Autodesk Fusion 360 part; units mm, degrees
(part 7 of 8)
  line L1736 (-325.3503, 148.8501) -> (-322.3503, 148.8501)
  line L1737 (-322.3503, 148.8501) -> (-322.3503, 151.8501)
  line L1738 (-322.3503, 151.8501) -> (-325.3503, 151.8501)
  line L1739 (-325.3503, 151.8501) -> (-325.3503, 154.8501)
  line L1740 (-325.3503, 154.8501) -> (-322.3503, 154.8501)
  line L1741 (-322.3503, 154.8501) -> (-322.3503, 157.8501)
  line L1742 (-322.3503, 157.8501) -> (-325.3503, 157.8501)
  line L1743 (-325.3503, 157.8501) -> (-325.3503, 160.8501)
  line L1744 (-325.3503, 160.8501) -> (-322.3503, 160.8501)
  line L1745 (-322.3503, 160.8501) -> (-322.3503, 163.8501)
  line L1746 (-322.3503, 163.8501) -> (-325.3503, 163.8501)
  line L1747 (-325.3503, 163.8501) -> (-325.3503, 166.8501)
  line L1748 (-325.3503, 166.8501) -> (-322.3503, 166.8501)
  line L1749 (-322.3503, 166.8501) -> (-322.3503, 169.8501)
  line L1750 (-322.3503, 169.8501) -> (-325.3503, 169.8501)
  line L1751 (-325.3503, 169.8501) -> (-325.3503, 172.8501)
  line L1752 (-325.3503, 172.8501) -> (-322.3503, 172.8501)
  line L1753 (-322.3503, 172.8501) -> (-322.3503, 176.6001)
  line L1754 (-322.3503, 176.6001) -> (-325.3503, 176.6001)
  line L1755 (-325.3503, 176.6001) -> (-325.3503, 177.3501)
  line L1756 (-325.3503, 177.3501) -> (-327.1003, 177.3501)
  line L1757 (-327.1003, 177.3501) -> (-327.1003, 180.3501)
  line L1758 (-327.1003, 180.3501) -> (-331.8503, 180.3501)
  line L1759 (-331.8503, 180.3501) -> (-331.8503, 177.3501)
  line L1760 (-331.8503, 177.3501) -> (-334.8503, 177.3501)
  line L1761 (-334.8503, 177.3501) -> (-334.8503, 180.3501)
  line L1762 (-334.8503, 180.3501) -> (-337.8503, 180.3501)
  line L1763 (-337.8503, 180.3501) -> (-337.8503, 177.3501)
  line L1764 (-337.8503, 177.3501) -> (-340.8503, 177.3501)
  line L1765 (-340.8503, 177.3501) -> (-340.8503, 180.3501)
  line L1766 (-340.8503, 180.3501) -> (-343.8503, 180.3501)
  line L1767 (-343.8503, 180.3501) -> (-343.8503, 177.3501)
  line L1768 (-343.8503, 177.3501) -> (-346.8503, 177.3501)
  line L1769 (-346.8503, 177.3501) -> (-346.8503, 180.3501)
  line L1770 (-346.8503, 180.3501) -> (-349.8503, 180.3501)
  line L1771 (-349.8503, 180.3501) -> (-349.8503, 177.3501)
  line L1772 (-349.8503, 177.3501) -> (-352.8503, 177.3501)
  line L1773 (-352.8503, 177.3501) -> (-352.8503, 180.3501)
  line L1774 (-352.8503, 180.3501) -> (-355.8503, 180.3501)
  line L1775 (-355.8503, 180.3501) -> (-355.8503, 177.3501)
  line L1776 (-355.8503, 177.3501) -> (-358.8503, 177.3501)
  line L1777 (-358.8503, 177.3501) -> (-358.8503, 180.3501)
  line L1778 (-358.8503, 180.3501) -> (-361.8503, 180.3501)
  line L1779 (-361.8503, 180.3501) -> (-361.8503, 177.3501)
  line L1780 (-361.8503, 177.3501) -> (-364.8503, 177.3501)
  line L1781 (-364.8503, 177.3501) -> (-364.8503, 180.3501)
  line L1782 (-364.8503, 180.3501) -> (-367.8503, 180.3501)
  line L1783 (-367.8503, 180.3501) -> (-367.8503, 177.3501)
  line L1784 (-367.8503, 177.3501) -> (-370.8503, 177.3501)
  line L1785 (-370.8503, 177.3501) -> (-370.8503, 180.3501)
  line L1786 (-370.8503, 180.3501) -> (-373.8503, 180.3501)
  line L1787 (-373.8503, 180.3501) -> (-373.8503, 177.3501)
  line L1788 (-373.8503, 177.3501) -> (-376.8503, 177.3501)
  line L1789 (-376.8503, 177.3501) -> (-376.8503, 180.3501)
  line L1790 (-376.8503, 180.3501) -> (-379.8503, 180.3501)
  line L1791 (-379.8503, 180.3501) -> (-379.8503, 177.3501)
  line L1792 (-379.8503, 177.3501) -> (-382.8503, 177.3501)
  line L1793 (-382.8503, 177.3501) -> (-382.8503, 180.3501)
  line L1794 (-382.8503, 180.3501) -> (-385.8503, 180.3501)
  line L1795 (-385.8503, 180.3501) -> (-385.8503, 177.3501)
  line L1796 (-385.8503, 177.3501) -> (-388.8503, 177.3501)
  line L1797 (-388.8503, 177.3501) -> (-388.8503, 180.3501)
  line L1798 (-388.8503, 180.3501) -> (-391.8503, 180.3501)
  line L1799 (-391.8503, 180.3501) -> (-391.8503, 177.3501)
  line L1800 (-391.8503, 177.3501) -> (-394.8503, 177.3501)
  line L1801 (-394.8503, 177.3501) -> (-394.8503, 180.3501)
  line L1802 (-394.8503, 180.3501) -> (-397.8503, 180.3501)
  line L1803 (-397.8503, 180.3501) -> (-397.8503, 177.3501)
  line L1804 (-397.8503, 177.3501) -> (-400.8503, 177.3501)
  line L1805 (-400.8503, 177.3501) -> (-400.8503, 180.3501)
  line L1806 (-400.8503, 180.3501) -> (-403.8503, 180.3501)
  line L1807 (-403.8503, 180.3501) -> (-403.8503, 177.3501)
  line L1808 (-403.8503, 177.3501) -> (-406.8503, 177.3501)
  line L1809 (-406.8503, 177.3501) -> (-406.8503, 180.3501)
  line L1810 (-406.8503, 180.3501) -> (-409.8503, 180.3501)
  line L1811 (-409.8503, 180.3501) -> (-409.8503, 177.3501)
  line L1812 (-409.8503, 177.3501) -> (-412.8503, 177.3501)
  line L1813 (-412.8503, 177.3501) -> (-412.8503, 180.3501)
  line L1814 (-412.8503, 180.3501) -> (-415.8503, 180.3501)
  line L1815 (-415.8503, 180.3501) -> (-415.8503, 177.3501)
  line L1816 (-415.8503, 177.3501) -> (-418.8503, 177.3501)
  line L1817 (-418.8503, 177.3501) -> (-418.8503, 180.3501)
  line L1818 (-418.8503, 180.3501) -> (-421.8503, 180.3501)
  line L1819 (-421.8503, 180.3501) -> (-421.8503, 177.3501)
  line L1820 (-421.8503, 177.3501) -> (-424.8503, 177.3501)
  line L1821 (-424.8503, 177.3501) -> (-424.8503, 180.3501)
  line L1822 (-424.8503, 180.3501) -> (-427.8504, 180.3501)
  line L1823 (-427.8504, 180.3501) -> (-427.8504, 177.3501)
  line L1824 (-427.8504, 177.3501) -> (-430.8504, 177.3501)
  line L1825 (-430.8504, 177.3501) -> (-430.8504, 180.3501)
  line L1826 (-430.8504, 180.3501) -> (-433.8504, 180.3501)
  line L1827 (-433.8504, 180.3501) -> (-433.8504, 177.3501)
  line L1828 (-433.8504, 177.3501) -> (-436.8504, 177.3501)
  line L1829 (-436.8504, 177.3501) -> (-436.8504, 180.3501)
  line L1830 (-436.8504, 180.3501) -> (-439.8504, 180.3501)
  line L1831 (-439.8504, 180.3501) -> (-439.8504, 177.3501)
  line L1832 (-439.8504, 177.3501) -> (-442.8504, 177.3501)
  line L1833 (-442.8504, 177.3501) -> (-442.8504, 180.3501)
  line L1834 (-442.8504, 180.3501) -> (-445.8504, 180.3501)
  line L1835 (-445.8504, 180.3501) -> (-445.8504, 177.3501)
  line L1836 (-445.8504, 177.3501) -> (-448.8504, 177.3501)
  line L1837 (-448.8504, 177.3501) -> (-448.8504, 180.3501)
  line L1838 (-448.8504, 180.3501) -> (-451.8504, 180.3501)
  line L1839 (-451.8504, 180.3501) -> (-451.8504, 177.3501)
  line L1840 (-451.8504, 177.3501) -> (-454.8504, 177.3501)
  line L1841 (-454.8504, 177.3501) -> (-454.8504, 180.3501)
  line L1842 (-454.8504, 180.3501) -> (-457.8504, 180.3501)
  line L1843 (-457.8504, 180.3501) -> (-457.8504, 177.3501)
  line L1844 (-457.8504, 177.3501) -> (-460.8504, 177.3501)
  line L1845 (-460.8504, 177.3501) -> (-460.8504, 180.3501)
  line L1846 (-460.8504, 180.3501) -> (-463.8504, 180.3501)
  line L1847 (-463.8504, 180.3501) -> (-463.8504, 177.3501)
  line L1848 (-463.8504, 177.3501) -> (-466.8504, 177.3501)
  line L1849 (-466.8504, 177.3501) -> (-466.8504, 180.3501)
  line L1850 (-466.8504, 180.3501) -> (-469.8504, 180.3501)
  line L1851 (-469.8504, 180.3501) -> (-469.8504, 177.3501)
  line L1852 (-469.8504, 177.3501) -> (-472.8504, 177.3501)
  line L1853 (-472.8504, 177.3501) -> (-472.8504, 180.3501)
  line L1854 (-472.8504, 180.3501) -> (-475.8504, 180.3501)
  line L1855 (-475.8504, 180.3501) -> (-475.8504, 177.3501)
  line L1856 (-475.8504, 177.3501) -> (-478.8504, 177.3501)
  line L1857 (-478.8504, 177.3501) -> (-478.8504, 180.3501)
  line L1858 (-478.8504, 180.3501) -> (-481.8504, 180.3501)
  line L1859 (-481.8504, 180.3501) -> (-481.8504, 177.3501)
  line L1860 (-481.8504, 177.3501) -> (-484.8504, 177.3501)
  line L1861 (-484.8504, 177.3501) -> (-484.8504, 180.3501)
  line L1862 (-484.8504, 180.3501) -> (-487.8504, 180.3501)
  line L1863 (-487.8504, 180.3501) -> (-487.8504, 177.3501)
  line L1864 (-487.8504, 177.3501) -> (-490.8504, 177.3501)
  line L1865 (-490.8504, 177.3501) -> (-490.8504, 180.3501)
  line L1866 (-490.8504, 180.3501) -> (-493.8504, 180.3501)
  line L1867 (-493.8504, 180.3501) -> (-493.8504, 177.3501)
  line L1868 (-493.8504, 177.3501) -> (-496.8504, 177.3501)
  line L1869 (-496.8504, 177.3501) -> (-496.8504, 180.3501)
  line L1870 (-496.8504, 180.3501) -> (-499.8504, 180.3501)
  line L1871 (-499.8504, 180.3501) -> (-499.8504, 177.3501)
  line L1872 (-499.8504, 177.3501) -> (-502.8504, 177.3501)
  line L1873 (-502.8504, 177.3501) -> (-502.8504, 180.3501)
  line L1874 (-502.8504, 180.3501) -> (-505.8504, 180.3501)
  line L1875 (-505.8504, 180.3501) -> (-505.8504, 177.3501)
  line L1876 (-505.8504, 177.3501) -> (-508.8504, 177.3501)
  line L1877 (-508.8504, 177.3501) -> (-508.8504, 180.3501)
  line L1878 (-508.8504, 180.3501) -> (-511.8504, 180.3501)
  line L1879 (-511.8504, 180.3501) -> (-511.8504, 177.3501)
  line L1880 (-511.8504, 177.3501) -> (-514.8504, 177.3501)
  line L1881 (-514.8504, 177.3501) -> (-514.8504, 180.3501)
  line L1882 (-514.8504, 180.3501) -> (-517.8504, 180.3501)
  line L1883 (-517.8504, 180.3501) -> (-517.8504, 177.3501)
  line L1884 (-517.8504, 177.3501) -> (-520.8504, 177.3501)
  line L1885 (-520.8504, 177.3501) -> (-520.8504, 180.3501)
  line L1886 (-520.8504, 180.3501) -> (-523.8504, 180.3501)
  line L1887 (-523.8504, 180.3501) -> (-523.8504, 177.3501)
  line L1888 (-523.8504, 177.3501) -> (-526.8504, 177.3501)
  line L1889 (-526.8504, 177.3501) -> (-526.8504, 180.3501)
  line L1890 (-526.8504, 180.3501) -> (-529.8504, 180.3501)
  line L1891 (-529.8504, 180.3501) -> (-529.8504, 177.3501)
  line L1892 (-529.8504, 177.3501) -> (-532.8504, 177.3501)
  line L1893 (-532.8504, 177.3501) -> (-532.8504, 180.3501)
  line L1894 (-532.8504, 180.3501) -> (-535.8504, 180.3501)
  line L1895 (-535.8504, 180.3501) -> (-535.8504, 177.3501)
  line L1896 (-535.8504, 177.3501) -> (-538.8504, 177.3501)
  line L1897 (-538.8504, 177.3501) -> (-538.8504, 180.3501)
  line L1898 (-538.8504, 180.3501) -> (-541.8504, 180.3501)
  line L1899 (-541.8504, 180.3501) -> (-541.8504, 177.3501)
  line L1900 (-541.8504, 177.3501) -> (-544.8504, 177.3501)
  line L1901 (-544.8504, 177.3501) -> (-544.8504, 180.3501)
  line L1902 (-544.8504, 180.3501) -> (-547.8505, 180.3501)
  line L1903 (-547.8505, 180.3501) -> (-547.8505, 177.3501)
  line L1904 (-547.8505, 177.3501) -> (-550.8505, 177.3501)
  line L1905 (-550.8505, 177.3501) -> (-550.8505, 180.3501)
  line L1906 (-550.8505, 180.3501) -> (-553.8505, 180.3501)
  line L1907 (-553.8505, 180.3501) -> (-553.8505, 177.3501)
  line L1908 (-553.8505, 177.3501) -> (-556.8505, 177.3501)
  line L1909 (-556.8505, 177.3501) -> (-556.8505, 180.3501)
  line L1910 (-556.8505, 180.3501) -> (-559.8505, 180.3501)
  line L1911 (-559.8505, 180.3501) -> (-559.8505, 177.3501)
  line L1912 (-559.8505, 177.3501) -> (-562.8505, 177.3501)
  line L1913 (-562.8505, 177.3501) -> (-562.8505, 180.3501)
  line L1914 (-562.8505, 180.3501) -> (-565.8505, 180.3501)
  line L1915 (-565.8505, 180.3501) -> (-565.8505, 177.3501)
  line L1916 (-565.8505, 177.3501) -> (-568.8505, 177.3501)
  line L1917 (-568.8505, 177.3501) -> (-568.8505, 180.3501)
  line L1918 (-568.8505, 180.3501) -> (-571.8505, 180.3501)
  line L1919 (-571.8505, 180.3501) -> (-571.8505, 177.3501)
  line L1920 (-571.8505, 177.3501) -> (-574.8505, 177.3501)
  line L1921 (-574.8505, 177.3501) -> (-574.8505, 180.3501)
  line L1922 (-574.8505, 180.3501) -> (-577.8505, 180.3501)
  line L1923 (-577.8505, 180.3501) -> (-577.8505, 177.3501)
  line L1924 (-577.8505, 177.3501) -> (-580.8505, 177.3501)
  line L1925 (-580.8505, 177.3501) -> (-580.8505, 180.3501)
  line L1926 (-580.8505, 180.3501) -> (-583.8505, 180.3501)
  line L1927 (-583.8505, 180.3501) -> (-583.8505, 177.3501)
  line L1928 (-583.8505, 177.3501) -> (-586.8505, 177.3501)
  line L1929 (-586.8505, 177.3501) -> (-586.8505, 180.3501)
  line L1930 (-586.8505, 180.3501) -> (-589.8505, 180.3501)
  line L1931 (-589.8505, 180.3501) -> (-589.8505, 177.3501)
  line L1932 (-589.8505, 177.3501) -> (-592.8505, 177.3501)
  line L1933 (-592.8505, 177.3501) -> (-592.8505, 180.3501)
  line L1934 (-592.8505, 180.3501) -> (-595.8505, 180.3501)
  line L1935 (-595.8505, 180.3501) -> (-595.8505, 177.3501)
  line L1936 (-595.8505, 177.3501) -> (-598.8505, 177.3501)
  line L1937 (-598.8505, 177.3501) -> (-598.8505, 180.3501)
  line L1938 (-598.8505, 180.3501) -> (-601.8505, 180.3501)
  line L1939 (-601.8505, 180.3501) -> (-601.8505, 177.3501)
  line L1940 (-601.8505, 177.3501) -> (-604.8505, 177.3501)
  line L1941 (-604.8505, 177.3501) -> (-604.8505, 180.3501)
  line L1942 (-604.8505, 180.3501) -> (-607.8505, 180.3501)
  line L1943 (-607.8505, 180.3501) -> (-607.8505, 177.3501)
  line L1944 (-607.8505, 177.3501) -> (-610.8505, 177.3501)
  line L1945 (-610.8505, 177.3501) -> (-610.8505, 180.3501)
  line L1946 (-610.8505, 180.3501) -> (-613.8505, 180.3501)
  line L1947 (-613.8505, 180.3501) -> (-613.8505, 177.3501)
  line L1948 (-613.8505, 177.3501) -> (-616.8505, 177.3501)
  line L1949 (-616.8505, 177.3501) -> (-616.8505, 180.3501)
  line L1950 (-616.8505, 180.3501) -> (-619.8505, 180.3501)
  line L1951 (-619.8505, 180.3501) -> (-619.8505, 177.3501)
  line L1952 (-619.8505, 177.3501) -> (-622.8505, 177.3501)
  line L1953 (-622.8505, 177.3501) -> (-622.8505, 180.3501)
  line L1954 (-622.8505, 180.3501) -> (-625.8505, 180.3501)
  line L1955 (-625.8505, 180.3501) -> (-625.8505, 177.3501)
  line L1956 (-625.8505, 177.3501) -> (-628.8505, 177.3501)
  line L1957 (-628.8505, 177.3501) -> (-628.8505, 180.3501)
  line L1958 (-628.8505, 180.3501) -> (-633.6005, 180.3501)
  line L1959 (-633.6005, 180.3501) -> (-633.6005, 177.3501)
  line L1960 (-633.6005, 177.3501) -> (-635.3505, 177.3501)
  line L1961 (-635.3505, 177.3501) -> (-635.3505, 176.6001)
  line L1962 (-635.3505, 176.6001) -> (-638.3505, 176.6001)
  line L1963 (-638.3505, 176.6001) -> (-638.3505, 172.8501)
  line L1964 (-638.3505, 172.8501) -> (-635.3505, 172.8501)
  line L1965 (-635.3505, 172.8501) -> (-635.3505, 169.8501)
  line L1966 (-635.3505, 169.8501) -> (-638.3505, 169.8501)
  line L1967 (-638.3505, 169.8501) -> (-638.3505, 166.8501)
  line L1968 (-638.3505, 166.8501) -> (-635.3505, 166.8501)
  line L1969 (-635.3505, 166.8501) -> (-635.3505, 163.8501)
  line L1970 (-635.3505, 163.8501) -> (-638.3505, 163.8501)
  line L1971 (-638.3505, 163.8501) -> (-638.3505, 160.8501)
  line L1972 (-638.3505, 160.8501) -> (-635.3505, 160.8501)
  line L1973 (-635.3505, 160.8501) -> (-635.3505, 157.8501)
  line L1974 (-635.3505, 157.8501) -> (-638.3505, 157.8501)
  line L1975 (-638.3505, 157.8501) -> (-638.3505, 154.8501)
  line L1976 (-638.3505, 154.8501) -> (-635.3505, 154.8501)
  line L1977 (-635.3505, 154.8501) -> (-635.3505, 151.8501)
  line L1978 (-635.3505, 151.8501) -> (-638.3505, 151.8501)
  line L1979 (-638.3505, 151.8501) -> (-638.3505, 148.8501)
  line L1980 (-638.3505, 148.8501) -> (-635.3505, 148.8501)
  line L1981 (-635.3505, 148.8501) -> (-635.3505, 145.8501)
  line L1982 (-635.3505, 145.8501) -> (-638.3505, 145.8501)
  line L1983 (-638.3505, 145.8501) -> (-638.3505, 142.8501)
  line L1984 (-638.3505, 142.8501) -> (-635.3505, 142.8501)
  line L1985 (-635.3505, 142.8501) -> (-635.3505, 139.8501)
  line L1986 (-635.3505, 139.8501) -> (-638.3505, 139.8501)
  line L1987 (-638.3505, 139.8501) -> (-638.3505, 136.8501)
  line L1988 (-638.3505, 136.8501) -> (-635.3505, 136.8501)
  line L1989 (-635.3505, 136.8501) -> (-635.3505, 133.8501)
  line L1990 (-635.3505, 133.8501) -> (-638.3505, 133.8501)
  line L1991 (-638.3505, 133.8501) -> (-638.3505, 130.8501)
  line L1992 (-638.3505, 130.8501) -> (-635.3505, 130.8501)
  line L1993 (-635.3505, 130.8501) -> (-635.3505, 127.8501)
  line L1994 (-635.3505, 127.8501) -> (-638.3505, 127.8501)
  line L1995 (-638.3505, 127.8501) -> (-638.3505, 124.8501)
  line L1996 (-638.3505, 124.8501) -> (-635.3505, 124.8501)
  line L1997 (-635.3505, 124.8501) -> (-635.3505, 121.8501)
  line L1998 (-635.3505, 121.8501) -> (-638.3505, 121.8501)
  line L1999 (-638.3505, 121.8501) -> (-638.3505, 118.8501)
  line L2000 (-638.3505, 118.8501) -> (-635.3505, 118.8501)
  line L2001 (-635.3505, 118.8501) -> (-635.3505, 115.8501)
  line L2002 (-635.3505, 115.8501) -> (-638.3505, 115.8501)
  line L2003 (-638.3505, 115.8501) -> (-638.3505, 112.8501)
  line L2004 (-638.3505, 112.8501) -> (-635.3505, 112.8501)
  line L2005 (-635.3505, 112.8501) -> (-635.3505, 109.8501)
  line L2006 (-635.3505, 109.8501) -> (-638.3505, 109.8501)
  line L2007 (-638.3505, 109.8501) -> (-638.3505, 106.8501)
  line L2008 (-638.3505, 106.8501) -> (-635.3505, 106.8501)
  line L2009 (-635.3505, 106.8501) -> (-635.3505, 103.8501)
  line L2010 (-635.3505, 103.8501) -> (-638.3505, 103.8501)
  line L2011 (-638.3505, 103.8501) -> (-638.3505, 100.8501)
  line L2012 (-638.3505, 100.8501) -> (-635.3505, 100.8501)
  line L2013 (-635.3505, 100.8501) -> (-635.3505, 97.8501)
  line L2014 (-635.3505, 97.8501) -> (-638.3505, 97.8501)
  line L2015 (-638.3505, 97.8501) -> (-638.3505, 94.8501)
  line L2016 (-638.3505, 94.8501) -> (-635.3505, 94.8501)
  line L2017 (-635.3505, 94.8501) -> (-635.3505, 91.8501)
  line L2018 (-635.3505, 91.8501) -> (-638.3505, 91.8501)
  line L2019 (-638.3505, 91.8501) -> (-638.3505, 88.8501)
  line L2020 (-638.3505, 88.8501) -> (-635.3505, 88.8501)
  line L2021 (-635.3505, 88.8501) -> (-635.3505, 85.8501)
  line L2022 (-635.3505, 85.8501) -> (-638.3505, 85.8501)
  line L2023 (-638.3505, 85.8501) -> (-638.3505, 82.8501)
  line L2024 (-638.3505, 82.8501) -> (-635.3505, 82.8501)
  line L2025 (-635.3505, 82.8501) -> (-635.3505, 79.8501)
  line L2026 (-635.3505, 79.8501) -> (-638.3505, 79.8501)
  line L2027 (-638.3505, 79.8501) -> (-638.3505, 76.8501)
  line L2028 (-638.3505, 76.8501) -> (-635.3505, 76.8501)
  line L2029 (-635.3505, 76.8501) -> (-635.3505, 73.8501)
  line L2030 (-635.3505, 73.8501) -> (-638.3505, 73.8501)
  line L2031 (-638.3505, 73.8501) -> (-638.3505, 70.8501)
  line L2032 (-638.3505, 70.8501) -> (-635.3505, 70.8501)
  line L2033 (-635.3505, 70.8501) -> (-635.3505, 67.8501)
  line L2034 (-635.3505, 67.8501) -> (-638.3505, 67.8501)
  line L2035 (-638.3505, 67.8501) -> (-638.3505, 64.8501)
  line L2036 (-638.3505, 64.8501) -> (-635.3505, 64.8501)
  line L2037 (-635.3505, 64.8501) -> (-635.3505, 61.8501)
  line L2038 (-635.3505, 61.8501) -> (-638.3505, 61.8501)
  line L2039 (-638.3505, 61.8501) -> (-638.3505, 58.85)
  line L2040 (-638.3505, 58.85) -> (-635.3505, 58.85)
  line L2041 (-635.3505, 58.85) -> (-635.3505, 55.85)
  line L2042 (-635.3505, 55.85) -> (-638.3505, 55.85)
  line L2043 (-638.3505, 55.85) -> (-638.3505, 52.85)
  line L2044 (-638.3505, 52.85) -> (-635.3505, 52.85)
  line L2045 (-635.3505, 52.85) -> (-635.3505, 49.85)
  line L2046 (-635.3505, 49.85) -> (-638.3505, 49.85)
  line L2047 (-638.3505, 49.85) -> (-638.3505, 46.85)
  line L2048 (-638.3505, 46.85) -> (-635.3505, 46.85)
  line L2049 (-635.3505, 46.85) -> (-635.3505, 43.85)
  line L2050 (-635.3505, 43.85) -> (-638.3505, 43.85)
  line L2051 (-638.3505, 43.85) -> (-638.3505, 40.85)
  line L2052 (-638.3505, 40.85) -> (-635.3505, 40.85)
  line L2053 (-635.3505, 40.85) -> (-635.3505, 37.85)
  line L2054 (-635.3505, 37.85) -> (-638.3505, 37.85)
  line L2055 (-638.3505, 37.85) -> (-638.3505, 34.85)
  line L2056 (-638.3505, 34.85) -> (-635.3505, 34.85)
  line L2057 (-635.3505, 34.85) -> (-635.3505, 31.85)
  line L2058 (-635.3505, 31.85) -> (-638.3505, 31.85)
  line L2059 (-638.3505, 31.85) -> (-638.3505, 28.1)
  line L2060 (-638.3505, 28.1) -> (-635.3505, 28.1)
  line L2061 (-635.3505, 28.1) -> (-635.3505, 27.35)
  line L2062 (-635.3505, 27.35) -> (-633.6005, 27.35)
  line L2063 (-633.6005, 27.35) -> (-633.6005, 24.35)
  line L2064 (-633.6005, 24.35) -> (-628.8505, 24.35)
  line L2065 (-628.8505, 24.35) -> (-628.8505, 27.35)
  line L2066 (-628.8505, 27.35) -> (-625.8505, 27.35)
  line L2067 (-625.8505, 27.35) -> (-625.8505, 24.35)
  line L2068 (-625.8505, 24.35) -> (-622.8505, 24.35)
  line L2069 (-622.8505, 24.35) -> (-622.8505, 27.35)
  line L2070 (-622.8505, 27.35) -> (-619.8505, 27.35)
  line L2071 (-619.8505, 27.35) -> (-619.8505, 24.35)
  line L2072 (-619.8505, 24.35) -> (-616.8505, 24.35)
  line L2073 (-616.8505, 24.35) -> (-616.8505, 27.35)
  line L2074 (-616.8505, 27.35) -> (-613.8505, 27.35)
  line L2075 (-613.8505, 27.35) -> (-613.8505, 24.35)
  line L2076 (-613.8505, 24.35) -> (-610.8505, 24.35)
  line L2077 (-610.8505, 24.35) -> (-610.8505, 27.35)
  line L2078 (-610.8505, 27.35) -> (-607.8505, 27.35)
  line L2079 (-607.8505, 27.35) -> (-607.8505, 24.35)
  line L2080 (-607.8505, 24.35) -> (-604.8505, 24.35)
  line L2081 (-604.8505, 24.35) -> (-604.8505, 27.35)
  line L2082 (-604.8505, 27.35) -> (-601.8505, 27.35)
  line L2083 (-601.8505, 27.35) -> (-601.8505, 24.35)
  line L2084 (-601.8505, 24.35) -> (-598.8505, 24.35)
  line L2085 (-598.8505, 24.35) -> (-598.8505, 27.35)
  line L2086 (-598.8505, 27.35) -> (-595.8505, 27.35)
  line L2087 (-595.8505, 27.35) -> (-595.8505, 24.35)
  line L2088 (-595.8505, 24.35) -> (-592.8505, 24.35)
  line L2089 (-592.8505, 24.35) -> (-592.8505, 27.35)
  line L2090 (-592.8505, 27.35) -> (-589.8505, 27.35)
  line L2091 (-589.8505, 27.35) -> (-589.8505, 24.35)
  line L2092 (-589.8505, 24.35) -> (-586.8505, 24.35)
  line L2093 (-586.8505, 24.35) -> (-586.8505, 27.35)
  line L2094 (-586.8505, 27.35) -> (-583.8505, 27.35)
  line L2095 (-583.8505, 27.35) -> (-583.8505, 24.35)
  line L2096 (-583.8505, 24.35) -> (-580.8505, 24.35)
  line L2097 (-580.8505, 24.35) -> (-580.8505, 27.35)
  line L2098 (-580.8505, 27.35) -> (-577.8505, 27.35)
  line L2099 (-577.8505, 27.35) -> (-577.8505, 24.35)
  line L2100 (-577.8505, 24.35) -> (-574.8505, 24.35)
  line L2101 (-574.8505, 24.35) -> (-574.8505, 27.35)
  line L2102 (-574.8505, 27.35) -> (-571.8505, 27.35)
  line L2103 (-571.8505, 27.35) -> (-571.8505, 24.35)
  line L2104 (-571.8505, 24.35) -> (-568.8505, 24.35)
  line L2105 (-568.8505, 24.35) -> (-568.8505, 27.35)
  line L2106 (-568.8505, 27.35) -> (-565.8505, 27.35)
  line L2107 (-565.8505, 27.35) -> (-565.8505, 24.35)
  line L2108 (-565.8505, 24.35) -> (-562.8505, 24.35)
  line L2109 (-562.8505, 24.35) -> (-562.8505, 27.35)
  line L2110 (-562.8505, 27.35) -> (-559.8505, 27.35)
  line L2111 (-559.8505, 27.35) -> (-559.8505, 24.35)
  line L2112 (-559.8505, 24.35) -> (-556.8505, 24.35)
  line L2113 (-556.8505, 24.35) -> (-556.8505, 27.35)
  line L2114 (-556.8505, 27.35) -> (-553.8505, 27.35)
  line L2115 (-553.8505, 27.35) -> (-553.8505, 24.35)
  line L2116 (-553.8505, 24.35) -> (-550.8505, 24.35)
  line L2117 (-550.8505, 24.35) -> (-550.8505, 27.35)
  line L2118 (-550.8505, 27.35) -> (-547.8505, 27.35)
  line L2119 (-547.8505, 27.35) -> (-547.8505, 24.35)
  line L2120 (-547.8505, 24.35) -> (-544.8504, 24.35)
  line L2121 (-544.8504, 24.35) -> (-544.8504, 27.35)
  line L2122 (-544.8504, 27.35) -> (-541.8504, 27.35)
  line L2123 (-541.8504, 27.35) -> (-541.8504, 24.35)
  line L2124 (-541.8504, 24.35) -> (-538.8504, 24.35)
  line L2125 (-538.8504, 24.35) -> (-538.8504, 27.35)
  line L2126 (-538.8504, 27.35) -> (-535.8504, 27.35)
  line L2127 (-535.8504, 27.35) -> (-535.8504, 24.35)
  line L2128 (-535.8504, 24.35) -> (-532.8504, 24.35)
  line L2129 (-532.8504, 24.35) -> (-532.8504, 27.35)
  line L2130 (-532.8504, 27.35) -> (-529.8504, 27.35)
  line L2131 (-529.8504, 27.35) -> (-529.8504, 24.35)
  line L2132 (-529.8504, 24.35) -> (-526.8504, 24.35)
  line L2133 (-526.8504, 24.35) -> (-526.8504, 27.35)
  line L2134 (-526.8504, 27.35) -> (-523.8504, 27.35)
  line L2135 (-523.8504, 27.35) -> (-523.8504, 24.35)
  line L2136 (-523.8504, 24.35) -> (-520.8504, 24.35)
  line L2137 (-520.8504, 24.35) -> (-520.8504, 27.35)
  line L2138 (-520.8504, 27.35) -> (-517.8504, 27.35)
  line L2139 (-517.8504, 27.35) -> (-517.8504, 24.35)
  line L2140 (-517.8504, 24.35) -> (-514.8504, 24.35)
  line L2141 (-514.8504, 24.35) -> (-514.8504, 27.35)
  line L2142 (-514.8504, 27.35) -> (-511.8504, 27.35)
  line L2143 (-511.8504, 27.35) -> (-511.8504, 24.35)
  line L2144 (-511.8504, 24.35) -> (-508.8504, 24.35)
  line L2145 (-508.8504, 24.35) -> (-508.8504, 27.35)
  line L2146 (-508.8504, 27.35) -> (-505.8504, 27.35)
  line L2147 (-505.8504, 27.35) -> (-505.8504, 24.35)
  line L2148 (-505.8504, 24.35) -> (-502.8504, 24.35)
  line L2149 (-502.8504, 24.35) -> (-502.8504, 27.35)
  line L2150 (-502.8504, 27.35) -> (-499.8504, 27.35)
  line L2151 (-499.8504, 27.35) -> (-499.8504, 24.35)
  line L2152 (-499.8504, 24.35) -> (-496.8504, 24.35)
  line L2153 (-496.8504, 24.35) -> (-496.8504, 27.35)
  line L2154 (-496.8504, 27.35) -> (-493.8504, 27.35)
  line L2155 (-493.8504, 27.35) -> (-493.8504, 24.35)
  line L2156 (-493.8504, 24.35) -> (-490.8504, 24.35)
  line L2157 (-490.8504, 24.35) -> (-490.8504, 27.35)
  line L2158 (-490.8504, 27.35) -> (-487.8504, 27.35)
  line L2159 (-487.8504, 27.35) -> (-487.8504, 24.35)
  line L2160 (-487.8504, 24.35) -> (-484.8504, 24.35)
  line L2161 (-484.8504, 24.35) -> (-484.8504, 27.35)
  line L2162 (-484.8504, 27.35) -> (-481.8504, 27.35)
  line L2163 (-481.8504, 27.35) -> (-481.8504, 24.35)
  line L2164 (-481.8504, 24.35) -> (-478.8504, 24.35)
  line L2165 (-478.8504, 24.35) -> (-478.8504, 27.35)
  line L2166 (-478.8504, 27.35) -> (-475.8504, 27.35)
  line L2167 (-475.8504, 27.35) -> (-475.8504, 24.35)
  line L2168 (-475.8504, 24.35) -> (-472.8504, 24.35)
  line L2169 (-472.8504, 24.35) -> (-472.8504, 27.35)
  line L2170 (-472.8504, 27.35) -> (-469.8504, 27.35)
  line L2171 (-469.8504, 27.35) -> (-469.8504, 24.35)
  line L2172 (-469.8504, 24.35) -> (-466.8504, 24.35)
  line L2173 (-466.8504, 24.35) -> (-466.8504, 27.35)
  line L2174 (-466.8504, 27.35) -> (-463.8504, 27.35)
  line L2175 (-463.8504, 27.35) -> (-463.8504, 24.35)
  line L2176 (-463.8504, 24.35) -> (-460.8504, 24.35)
  line L2177 (-460.8504, 24.35) -> (-460.8504, 27.35)
  line L2178 (-460.8504, 27.35) -> (-457.8504, 27.35)
  line L2179 (-457.8504, 27.35) -> (-457.8504, 24.35)
  line L2180 (-457.8504, 24.35) -> (-454.8504, 24.35)
  line L2181 (-454.8504, 24.35) -> (-454.8504, 27.35)
  line L2182 (-454.8504, 27.35) -> (-451.8504, 27.35)
  line L2183 (-451.8504, 27.35) -> (-451.8504, 24.35)
  line L2184 (-451.8504, 24.35) -> (-448.8504, 24.35)
  line L2185 (-448.8504, 24.35) -> (-448.8504, 27.35)
  line L2186 (-448.8504, 27.35) -> (-445.8504, 27.35)
  line L2187 (-445.8504, 27.35) -> (-445.8504, 24.35)
  line L2188 (-445.8504, 24.35) -> (-442.8504, 24.35)
  line L2189 (-442.8504, 24.35) -> (-442.8504, 27.35)
  line L2190 (-442.8504, 27.35) -> (-439.8504, 27.35)
  line L2191 (-439.8504, 27.35) -> (-439.8504, 24.35)
  line L2192 (-439.8504, 24.35) -> (-436.8504, 24.35)
  line L2193 (-436.8504, 24.35) -> (-436.8504, 27.35)
  line L2194 (-436.8504, 27.35) -> (-433.8504, 27.35)
  line L2195 (-433.8504, 27.35) -> (-433.8504, 24.35)
  line L2196 (-433.8504, 24.35) -> (-430.8504, 24.35)
  line L2197 (-430.8504, 24.35) -> (-430.8504, 27.35)
  line L2198 (-430.8504, 27.35) -> (-427.8504, 27.35)
  line L2199 (-427.8504, 27.35) -> (-427.8504, 24.35)
  line L2200 (-427.8504, 24.35) -> (-424.8503, 24.35)
  line L2201 (-424.8503, 24.35) -> (-424.8503, 27.35)
  line L2202 (-424.8503, 27.35) -> (-421.8503, 27.35)
  line L2203 (-421.8503, 27.35) -> (-421.8503, 24.35)
  line L2204 (-421.8503, 24.35) -> (-418.8503, 24.35)
  line L2205 (-418.8503, 24.35) -> (-418.8503, 27.35)
  line L2206 (-418.8503, 27.35) -> (-415.8503, 27.35)
  line L2207 (-415.8503, 27.35) -> (-415.8503, 24.35)
  line L2208 (-415.8503, 24.35) -> (-412.8503, 24.35)
  line L2209 (-412.8503, 24.35) -> (-412.8503, 27.35)
  line L2210 (-412.8503, 27.35) -> (-409.8503, 27.35)
  line L2211 (-409.8503, 27.35) -> (-409.8503, 24.35)
  line L2212 (-409.8503, 24.35) -> (-406.8503, 24.35)
  line L2213 (-406.8503, 24.35) -> (-406.8503, 27.35)
  line L2214 (-406.8503, 27.35) -> (-403.8503, 27.35)
  line L2215 (-403.8503, 27.35) -> (-403.8503, 24.35)
  line L2216 (-403.8503, 24.35) -> (-400.8503, 24.35)
  line L2217 (-400.8503, 24.35) -> (-400.8503, 27.35)
  line L2218 (-400.8503, 27.35) -> (-397.8503, 27.35)
  line L2219 (-397.8503, 27.35) -> (-397.8503, 24.35)
  line L2220 (-397.8503, 24.35) -> (-394.8503, 24.35)
  line L2221 (-394.8503, 24.35) -> (-394.8503, 27.35)
  line L2222 (-394.8503, 27.35) -> (-391.8503, 27.35)
  line L2223 (-391.8503, 27.35) -> (-391.8503, 24.35)
  line L2224 (-391.8503, 24.35) -> (-388.8503, 24.35)
  line L2225 (-388.8503, 24.35) -> (-388.8503, 27.35)
  line L2226 (-388.8503, 27.35) -> (-385.8503, 27.35)
  line L2227 (-385.8503, 27.35) -> (-385.8503, 24.35)
  line L2228 (-385.8503, 24.35) -> (-382.8503, 24.35)
  line L2229 (-382.8503, 24.35) -> (-382.8503, 27.35)
  line L2230 (-382.8503, 27.35) -> (-379.8503, 27.35)
  line L2231 (-379.8503, 27.35) -> (-379.8503, 24.35)
  line L2232 (-379.8503, 24.35) -> (-376.8503, 24.35)
  line L2233 (-376.8503, 24.35) -> (-376.8503, 27.35)
  line L2234 (-376.8503, 27.35) -> (-373.8503, 27.35)
  line L2235 (-373.8503, 27.35) -> (-373.8503, 24.35)
  line L2236 (-373.8503, 24.35) -> (-370.8503, 24.35)
  line L2237 (-370.8503, 24.35) -> (-370.8503, 27.35)
  line L2238 (-370.8503, 27.35) -> (-367.8503, 27.35)
  line L2239 (-367.8503, 27.35) -> (-367.8503, 24.35)
  line L2240 (-367.8503, 24.35) -> (-364.8503, 24.35)
  line L2241 (-364.8503, 24.35) -> (-364.8503, 27.35)
  line L2242 (-364.8503, 27.35) -> (-361.8503, 27.35)
  line L2243 (-361.8503, 27.35) -> (-361.8503, 24.35)
  line L2244 (-361.8503, 24.35) -> (-358.8503, 24.35)
  line L2245 (-358.8503, 24.35) -> (-358.8503, 27.35)
  line L2246 (-358.8503, 27.35) -> (-355.8503, 27.35)
  line L2247 (-355.8503, 27.35) -> (-355.8503, 24.35)
  line L2248 (-355.8503, 24.35) -> (-352.8503, 24.35)
  line L2249 (-352.8503, 24.35) -> (-352.8503, 27.35)
  line L2250 (-352.8503, 27.35) -> (-349.8503, 27.35)
  line L2251 (-349.8503, 27.35) -> (-349.8503, 24.35)
  line L2252 (-349.8503, 24.35) -> (-346.8503, 24.35)
  line L2253 (-346.8503, 24.35) -> (-346.8503, 27.35)
  line L2254 (-346.8503, 27.35) -> (-343.8503, 27.35)
  line L2255 (-343.8503, 27.35) -> (-343.8503, 24.35)
  line L2256 (-343.8503, 24.35) -> (-340.8503, 24.35)
  line L2257 (-340.8503, 24.35) -> (-340.8503, 27.35)
  line L2258 (-340.8503, 27.35) -> (-337.8503, 27.35)
  line L2259 (-337.8503, 27.35) -> (-337.8503, 24.35)
  line L2260 (-337.8503, 24.35) -> (-334.8503, 24.35)
  line L2261 (-334.8503, 24.35) -> (-334.8503, 27.35)
  line L2262 (-334.8503, 27.35) -> (-331.8503, 27.35)
  line L2263 (-331.8503, 27.35) -> (-331.8503, 24.35)
  line L2264 (-331.8503, 24.35) -> (-327.1003, 24.35)
  line L2265 (-327.1003, 24.35) -> (-327.1003, 27.35)
  line L2266 (-327.1003, 27.35) -> (-325.3503, 27.35)
  line L2267 (-325.3503, 27.35) -> (-325.3503, 28.1)
  line L2268 (-322.3503, 10.1) -> (-325.3503, 10.1)
  line L2269 (-325.3503, 10.1) -> (-325.3503, 13.85)
  line L2270 (-325.3503, 13.85) -> (-322.3503, 13.85)
  line L2271 (-322.3503, 13.85) -> (-322.3503, 16.85)
  line L2272 (-322.3503, 16.85) -> (-325.3503, 16.85)
  line L2273 (-325.3503, 16.85) -> (-325.3503, 20.6)
  line L2274 (-325.3503, 20.6) -> (-322.3503, 20.6)
  line L2275 (-322.3503, 20.6) -> (-322.3503, 24.35)
  line L2276 (-322.3503, 24.35) -> (-327.1003, 24.35)
  line L2277 (-327.1003, 24.35) -> (-327.1003, 21.35)
  line L2278 (-327.1003, 21.35) -> (-331.8503, 21.35)
  line L2279 (-331.8503, 21.35) -> (-331.8503, 24.35)
  line L2280 (-331.8503, 24.35) -> (-334.8503, 24.35)
  line L2281 (-334.8503, 24.35) -> (-334.8503, 21.35)
  line L2282 (-334.8503, 21.35) -> (-337.8503, 21.35)
  line L2283 (-337.8503, 21.35) -> (-337.8503, 24.35)
  line L2284 (-337.8503, 24.35) -> (-340.8503, 24.35)
  line L2285 (-340.8503, 24.35) -> (-340.8503, 21.35)
  line L2286 (-340.8503, 21.35) -> (-343.8503, 21.35)
  line L2287 (-343.8503, 21.35) -> (-343.8503, 24.35)
  line L2288 (-343.8503, 24.35) -> (-346.8503, 24.35)
  line L2289 (-346.8503, 24.35) -> (-346.8503, 21.35)
  line L2290 (-346.8503, 21.35) -> (-349.8503, 21.35)
  line L2291 (-349.8503, 21.35) -> (-349.8503, 24.35)
  line L2292 (-349.8503, 24.35) -> (-352.8503, 24.35)
  line L2293 (-352.8503, 24.35) -> (-352.8503, 21.35)
  line L2294 (-352.8503, 21.35) -> (-355.8503, 21.35)
  line L2295 (-355.8503, 21.35) -> (-355.8503, 24.35)
  line L2296 (-355.8503, 24.35) -> (-358.8503, 24.35)
  line L2297 (-358.8503, 24.35) -> (-358.8503, 21.35)
  line L2298 (-358.8503, 21.35) -> (-361.8503, 21.35)
  line L2299 (-361.8503, 21.35) -> (-361.8503, 24.35)
  line L2300 (-361.8503, 24.35) -> (-364.8503, 24.35)
  line L2301 (-364.8503, 24.35) -> (-364.8503, 21.35)
  line L2302 (-364.8503, 21.35) -> (-367.8503, 21.35)
  line L2303 (-367.8503, 21.35) -> (-367.8503, 24.35)
  line L2304 (-367.8503, 24.35) -> (-370.8503, 24.35)
  line L2305 (-370.8503, 24.35) -> (-370.8503, 21.35)
  line L2306 (-370.8503, 21.35) -> (-373.8503, 21.35)
  line L2307 (-373.8503, 21.35) -> (-373.8503, 24.35)
  line L2308 (-373.8503, 24.35) -> (-376.8503, 24.35)
  line L2309 (-376.8503, 24.35) -> (-376.8503, 21.35)
  line L2310 (-376.8503, 21.35) -> (-379.8503, 21.35)
  line L2311 (-379.8503, 21.35) -> (-379.8503, 24.35)
  line L2312 (-379.8503, 24.35) -> (-382.8503, 24.35)
  line L2313 (-382.8503, 24.35) -> (-382.8503, 21.35)
  line L2314 (-382.8503, 21.35) -> (-385.8503, 21.35)
  line L2315 (-385.8503, 21.35) -> (-385.8503, 24.35)
  line L2316 (-385.8503, 24.35) -> (-388.8503, 24.35)
  line L2317 (-388.8503, 24.35) -> (-388.8503, 21.35)
  line L2318 (-388.8503, 21.35) -> (-391.8503, 21.35)
  line L2319 (-391.8503, 21.35) -> (-391.8503, 24.35)
  line L2320 (-391.8503, 24.35) -> (-394.8503, 24.35)
  line L2321 (-394.8503, 24.35) -> (-394.8503, 21.35)
  line L2322 (-394.8503, 21.35) -> (-397.8503, 21.35)
  line L2323 (-397.8503, 21.35) -> (-397.8503, 24.35)
  line L2324 (-397.8503, 24.35) -> (-400.8503, 24.35)
  line L2325 (-400.8503, 24.35) -> (-400.8503, 21.35)
  line L2326 (-400.8503, 21.35) -> (-403.8503, 21.35)
  line L2327 (-403.8503, 21.35) -> (-403.8503, 24.35)
  line L2328 (-403.8503, 24.35) -> (-406.8503, 24.35)
  line L2329 (-406.8503, 24.35) -> (-406.8503, 21.35)
  line L2330 (-406.8503, 21.35) -> (-409.8503, 21.35)
  line L2331 (-409.8503, 21.35) -> (-409.8503, 24.35)
  line L2332 (-409.8503, 24.35) -> (-412.8503, 24.35)
  line L2333 (-412.8503, 24.35) -> (-412.8503, 21.35)
  line L2334 (-412.8503, 21.35) -> (-415.8503, 21.35)
  line L2335 (-415.8503, 21.35) -> (-415.8503, 24.35)
  line L2336 (-415.8503, 24.35) -> (-418.8503, 24.35)
  line L2337 (-418.8503, 24.35) -> (-418.8503, 21.35)
  line L2338 (-418.8503, 21.35) -> (-421.8503, 21.35)
  line L2339 (-421.8503, 21.35) -> (-421.8503, 24.35)
  line L2340 (-421.8503, 24.35) -> (-424.8503, 24.35)
  line L2341 (-424.8503, 24.35) -> (-424.8503, 21.35)
  line L2342 (-424.8503, 21.35) -> (-427.8504, 21.35)
  line L2343 (-427.8504, 21.35) -> (-427.8504, 24.35)
  line L2344 (-427.8504, 24.35) -> (-430.8504, 24.35)
  line L2345 (-430.8504, 24.35) -> (-430.8504, 21.35)
  line L2346 (-430.8504, 21.35) -> (-433.8504, 21.35)
  line L2347 (-433.8504, 21.35) -> (-433.8504, 24.35)
  line L2348 (-433.8504, 24.35) -> (-436.8504, 24.35)
  line L2349 (-436.8504, 24.35) -> (-436.8504, 21.35)
  line L2350 (-436.8504, 21.35) -> (-439.8504, 21.35)
  line L2351 (-439.8504, 21.35) -> (-439.8504, 24.35)
  line L2352 (-439.8504, 24.35) -> (-442.8504, 24.35)
  line L2353 (-442.8504, 24.35) -> (-442.8504, 21.35)
  line L2354 (-442.8504, 21.35) -> (-445.8504, 21.35)
  line L2355 (-445.8504, 21.35) -> (-445.8504, 24.35)
  line L2356 (-445.8504, 24.35) -> (-448.8504, 24.35)
  line L2357 (-448.8504, 24.35) -> (-448.8504, 21.35)
  line L2358 (-448.8504, 21.35) -> (-451.8504, 21.35)
  line L2359 (-451.8504, 21.35) -> (-451.8504, 24.35)
  line L2360 (-451.8504, 24.35) -> (-454.8504, 24.35)
  line L2361 (-454.8504, 24.35) -> (-454.8504, 21.35)
  line L2362 (-454.8504, 21.35) -> (-457.8504, 21.35)
  line L2363 (-457.8504, 21.35) -> (-457.8504, 24.35)
  line L2364 (-457.8504, 24.35) -> (-460.8504, 24.35)
  line L2365 (-460.8504, 24.35) -> (-460.8504, 21.35)
  line L2366 (-460.8504, 21.35) -> (-463.8504, 21.35)
  line L2367 (-463.8504, 21.35) -> (-463.8504, 24.35)
  line L2368 (-463.8504, 24.35) -> (-466.8504, 24.35)
  line L2369 (-466.8504, 24.35) -> (-466.8504, 21.35)
  line L2370 (-466.8504, 21.35) -> (-469.8504, 21.35)
  line L2371 (-469.8504, 21.35) -> (-469.8504, 24.35)
  line L2372 (-469.8504, 24.35) -> (-472.8504, 24.35)
  line L2373 (-472.8504, 24.35) -> (-472.8504, 21.35)
  line L2374 (-472.8504, 21.35) -> (-475.8504, 21.35)
  line L2375 (-475.8504, 21.35) -> (-475.8504, 24.35)
  line L2376 (-475.8504, 24.35) -> (-478.8504, 24.35)
  line L2377 (-478.8504, 24.35) -> (-478.8504, 21.35)
  line L2378 (-478.8504, 21.35) -> (-481.8504, 21.35)
  line L2379 (-481.8504, 21.35) -> (-481.8504, 24.35)
  line L2380 (-481.8504, 24.35) -> (-484.8504, 24.35)
  line L2381 (-484.8504, 24.35) -> (-484.8504, 21.35)
  line L2382 (-484.8504, 21.35) -> (-487.8504, 21.35)
  line L2383 (-487.8504, 21.35) -> (-487.8504, 24.35)
  line L2384 (-487.8504, 24.35) -> (-490.8504, 24.35)
  line L2385 (-490.8504, 24.35) -> (-490.8504, 21.35)
  line L2386 (-490.8504, 21.35) -> (-493.8504, 21.35)
  line L2387 (-493.8504, 21.35) -> (-493.8504, 24.35)
  line L2388 (-493.8504, 24.35) -> (-496.8504, 24.35)
  line L2389 (-496.8504, 24.35) -> (-496.8504, 21.35)
  line L2390 (-496.8504, 21.35) -> (-499.8504, 21.35)
  line L2391 (-499.8504, 21.35) -> (-499.8504, 24.35)
  line L2392 (-499.8504, 24.35) -> (-502.8504, 24.35)
  line L2393 (-502.8504, 24.35) -> (-502.8504, 21.35)
  line L2394 (-502.8504, 21.35) -> (-505.8504, 21.35)
  line L2395 (-505.8504, 21.35) -> (-505.8504, 24.35)
  line L2396 (-505.8504, 24.35) -> (-508.8504, 24.35)
  line L2397 (-508.8504, 24.35) -> (-508.8504, 21.35)
  line L2398 (-508.8504, 21.35) -> (-511.8504, 21.35)
  line L2399 (-511.8504, 21.35) -> (-511.8504, 24.35)
  line L2400 (-511.8504, 24.35) -> (-514.8504, 24.35)
  line L2401 (-514.8504, 24.35) -> (-514.8504, 21.35)
  line L2402 (-514.8504, 21.35) -> (-517.8504, 21.35)
  line L2403 (-517.8504, 21.35) -> (-517.8504, 24.35)
  line L2404 (-517.8504, 24.35) -> (-520.8504, 24.35)
  line L2405 (-520.8504, 24.35) -> (-520.8504, 21.35)
  line L2406 (-520.8504, 21.35) -> (-523.8504, 21.35)
  line L2407 (-523.8504, 21.35) -> (-523.8504, 24.35)
  line L2408 (-523.8504, 24.35) -> (-526.8504, 24.35)
  line L2409 (-526.8504, 24.35) -> (-526.8504, 21.35)
  line L2410 (-526.8504, 21.35) -> (-529.8504, 21.35)
  line L2411 (-529.8504, 21.35) -> (-529.8504, 24.35)
  line L2412 (-529.8504, 24.35) -> (-532.8504, 24.35)
  line L2413 (-532.8504, 24.35) -> (-532.8504, 21.35)
  line L2414 (-532.8504, 21.35) -> (-535.8504, 21.35)
  line L2415 (-535.8504, 21.35) -> (-535.8504, 24.35)
  line L2416 (-535.8504, 24.35) -> (-538.8504, 24.35)
  line L2417 (-538.8504, 24.35) -> (-538.8504, 21.35)
  line L2418 (-538.8504, 21.35) -> (-541.8504, 21.35)
  line L2419 (-541.8504, 21.35) -> (-541.8504, 24.35)
  line L2420 (-541.8504, 24.35) -> (-544.8504, 24.35)
  line L2421 (-544.8504, 24.35) -> (-544.8504, 21.35)
  line L2422 (-544.8504, 21.35) -> (-547.8505, 21.35)
  line L2423 (-547.8505, 21.35) -> (-547.8505, 24.35)
  line L2424 (-547.8505, 24.35) -> (-550.8505, 24.35)
  line L2425 (-550.8505, 24.35) -> (-550.8505, 21.35)
  line L2426 (-550.8505, 21.35) -> (-553.8505, 21.35)
  line L2427 (-553.8505, 21.35) -> (-553.8505, 24.35)
  line L2428 (-553.8505, 24.35) -> (-556.8505, 24.35)
  line L2429 (-556.8505, 24.35) -> (-556.8505, 21.35)
  line L2430 (-556.8505, 21.35) -> (-559.8505, 21.35)
  line L2431 (-559.8505, 21.35) -> (-559.8505, 24.35)
  line L2432 (-559.8505, 24.35) -> (-562.8505, 24.35)
  line L2433 (-562.8505, 24.35) -> (-562.8505, 21.35)
  line L2434 (-562.8505, 21.35) -> (-565.8505, 21.35)
  line L2435 (-565.8505, 21.35) -> (-565.8505, 24.35)
  line L2436 (-565.8505, 24.35) -> (-568.8505, 24.35)
  line L2437 (-568.8505, 24.35) -> (-568.8505, 21.35)
  line L2438 (-568.8505, 21.35) -> (-571.8505, 21.35)
  line L2439 (-571.8505, 21.35) -> (-571.8505, 24.35)
  line L2440 (-571.8505, 24.35) -> (-574.8505, 24.35)
  line L2441 (-574.8505, 24.35) -> (-574.8505, 21.35)
  line L2442 (-574.8505, 21.35) -> (-577.8505, 21.35)
  line L2443 (-577.8505, 21.35) -> (-577.8505, 24.35)
  line L2444 (-577.8505, 24.35) -> (-580.8505, 24.35)
  line L2445 (-580.8505, 24.35) -> (-580.8505, 21.35)
  line L2446 (-580.8505, 21.35) -> (-583.8505, 21.35)
  line L2447 (-583.8505, 21.35) -> (-583.8505, 24.35)
  line L2448 (-583.8505, 24.35) -> (-586.8505, 24.35)
  line L2449 (-586.8505, 24.35) -> (-586.8505, 21.35)
  line L2450 (-586.8505, 21.35) -> (-589.8505, 21.35)
  line L2451 (-589.8505, 21.35) -> (-589.8505, 24.35)
  line L2452 (-589.8505, 24.35) -> (-592.8505, 24.35)
  line L2453 (-592.8505, 24.35) -> (-592.8505, 21.35)
  line L2454 (-592.8505, 21.35) -> (-595.8505, 21.35)
  line L2455 (-595.8505, 21.35) -> (-595.8505, 24.35)
  line L2456 (-595.8505, 24.35) -> (-598.8505, 24.35)
  line L2457 (-598.8505, 24.35) -> (-598.8505, 21.35)
  line L2458 (-598.8505, 21.35) -> (-601.8505, 21.35)
  line L2459 (-601.8505, 21.35) -> (-601.8505, 24.35)
  line L2460 (-601.8505, 24.35) -> (-604.8505, 24.35)
  line L2461 (-604.8505, 24.35) -> (-604.8505, 21.35)
  line L2462 (-604.8505, 21.35) -> (-607.8505, 21.35)
  line L2463 (-607.8505, 21.35) -> (-607.8505, 24.35)
  line L2464 (-607.8505, 24.35) -> (-610.8505, 24.35)
  line L2465 (-610.8505, 24.35) -> (-610.8505, 21.35)
  line L2466 (-610.8505, 21.35) -> (-613.8505, 21.35)
  line L2467 (-613.8505, 21.35) -> (-613.8505, 24.35)
  line L2468 (-613.8505, 24.35) -> (-616.8505, 24.35)
  line L2469 (-616.8505, 24.35) -> (-616.8505, 21.35)
  line L2470 (-616.8505, 21.35) -> (-619.8505, 21.35)
  line L2471 (-619.8505, 21.35) -> (-619.8505, 24.35)
  line L2472 (-619.8505, 24.35) -> (-622.8505, 24.35)
  line L2473 (-622.8505, 24.35) -> (-622.8505, 21.35)
  line L2474 (-622.8505, 21.35) -> (-625.8505, 21.35)
  line L2475 (-625.8505, 21.35) -> (-625.8505, 24.35)
  line L2476 (-625.8505, 24.35) -> (-628.8505, 24.35)
  line L2477 (-628.8505, 24.35) -> (-628.8505, 21.35)
  line L2478 (-628.8505, 21.35) -> (-633.6005, 21.35)
  line L2479 (-633.6005, 21.35) -> (-633.6005, 24.35)
  line L2480 (-633.6005, 24.35) -> (-638.3505, 24.35)
  line L2481 (-638.3505, 24.35) -> (-638.3505, 20.6)
  line L2482 (-638.3505, 20.6) -> (-635.3505, 20.6)
  line L2483 (-635.3505, 20.6) -> (-635.3505, 16.85)
  line L2484 (-635.3505, 16.85) -> (-638.3505, 16.85)
  line L2485 (-638.3505, 16.85) -> (-638.3505, 13.85)
  line L2486 (-638.3505, 13.85) -> (-635.3505, 13.85)
  line L2487 (-635.3505, 13.85) -> (-635.3505, 10.1)
  line L2488 (-635.3505, 10.1) -> (-638.3505, 10.1)
  line L2489 (-638.3505, 10.1) -> (-638.3505, 6.35)
  line L2490 (-638.3505, 6.35) -> (-633.6005, 6.35)
  line L2491 (-633.6005, 6.35) -> (-633.6005, 9.35)
  line L2492 (-633.6005, 9.35) -> (-628.8505, 9.35)
  line L2493 (-628.8505, 9.35) -> (-628.8505, 6.35)
  line L2494 (-628.8505, 6.35) -> (-625.8505, 6.35)
  line L2495 (-625.8505, 6.35) -> (-625.8505, 9.35)
  line L2496 (-625.8505, 9.35) -> (-622.8505, 9.35)
  line L2497 (-622.8505, 9.35) -> (-622.8505, 6.35)
  line L2498 (-622.8505, 6.35) -> (-619.8505, 6.35)
  line L2499 (-619.8505, 6.35) -> (-619.8505, 9.35)
  line L2500 (-619.8505, 9.35) -> (-616.8505, 9.35)
  line L2501 (-616.8505, 9.35) -> (-616.8505, 6.35)
  line L2502 (-616.8505, 6.35) -> (-613.8505, 6.35)
  line L2503 (-613.8505, 6.35) -> (-613.8505, 9.35)
  line L2504 (-613.8505, 9.35) -> (-610.8505, 9.35)
  line L2505 (-610.8505, 9.35) -> (-610.8505, 6.35)
  line L2506 (-610.8505, 6.35) -> (-607.8505, 6.35)
  line L2507 (-607.8505, 6.35) -> (-607.8505, 9.35)
  line L2508 (-607.8505, 9.35) -> (-604.8505, 9.35)
  line L2509 (-604.8505, 9.35) -> (-604.8505, 6.35)
  line L2510 (-604.8505, 6.35) -> (-601.8505, 6.35)
  line L2511 (-601.8505, 6.35) -> (-601.8505, 9.35)
  line L2512 (-601.8505, 9.35) -> (-598.8505, 9.35)
  line L2513 (-598.8505, 9.35) -> (-598.8505, 6.35)
  line L2514 (-598.8505, 6.35) -> (-595.8505, 6.35)
  line L2515 (-595.8505, 6.35) -> (-595.8505, 9.35)
  line L2516 (-595.8505, 9.35) -> (-592.8505, 9.35)
  line L2517 (-592.8505, 9.35) -> (-592.8505, 6.35)
  line L2518 (-592.8505, 6.35) -> (-589.8505, 6.35)
  line L2519 (-589.8505, 6.35) -> (-589.8505, 9.35)
  line L2520 (-589.8505, 9.35) -> (-586.8505, 9.35)
  line L2521 (-586.8505, 9.35) -> (-586.8505, 6.35)
  line L2522 (-586.8505, 6.35) -> (-583.8505, 6.35)
  line L2523 (-583.8505, 6.35) -> (-583.8505, 9.35)
  line L2524 (-583.8505, 9.35) -> (-580.8505, 9.35)
  line L2525 (-580.8505, 9.35) -> (-580.8505, 6.35)
  line L2526 (-580.8505, 6.35) -> (-577.8505, 6.35)
  line L2527 (-577.8505, 6.35) -> (-577.8505, 9.35)
  line L2528 (-577.8505, 9.35) -> (-574.8505, 9.35)
  line L2529 (-574.8505, 9.35) -> (-574.8505, 6.35)
  line L2530 (-574.8505, 6.35) -> (-571.8505, 6.35)
  line L2531 (-571.8505, 6.35) -> (-571.8505, 9.35)
  line L2532 (-571.8505, 9.35) -> (-568.8505, 9.35)
  line L2533 (-568.8505, 9.35) -> (-568.8505, 6.35)
  line L2534 (-568.8505, 6.35) -> (-565.8505, 6.35)
  line L2535 (-565.8505, 6.35) -> (-565.8505, 9.35)
  line L2536 (-565.8505, 9.35) -> (-562.8505, 9.35)
  line L2537 (-562.8505, 9.35) -> (-562.8505, 6.35)
  line L2538 (-562.8505, 6.35) -> (-559.8505, 6.35)
  line L2539 (-559.8505, 6.35) -> (-559.8505, 9.35)
  line L2540 (-559.8505, 9.35) -> (-556.8505, 9.35)
  line L2541 (-556.8505, 9.35) -> (-556.8505, 6.35)
  line L2542 (-556.8505, 6.35) -> (-553.8505, 6.35)
  line L2543 (-553.8505, 6.35) -> (-553.8505, 9.35)
  line L2544 (-553.8505, 9.35) -> (-550.8505, 9.35)
  line L2545 (-550.8505, 9.35) -> (-550.8505, 6.35)
  line L2546 (-550.8505, 6.35) -> (-547.8505, 6.35)
  line L2547 (-547.8505, 6.35) -> (-547.8505, 9.35)
  line L2548 (-547.8505, 9.35) -> (-544.8504, 9.35)
  line L2549 (-544.8504, 9.35) -> (-544.8504, 6.35)
  line L2550 (-544.8504, 6.35) -> (-541.8504, 6.35)
  line L2551 (-541.8504, 6.35) -> (-541.8504, 9.35)
  line L2552 (-541.8504, 9.35) -> (-538.8504, 9.35)
  line L2553 (-538.8504, 9.35) -> (-538.8504, 6.35)
  line L2554 (-538.8504, 6.35) -> (-535.8504, 6.35)
  line L2555 (-535.8504, 6.35) -> (-535.8504, 9.35)
  line L2556 (-535.8504, 9.35) -> (-532.8504, 9.35)
  line L2557 (-532.8504, 9.35) -> (-532.8504, 6.35)
  line L2558 (-532.8504, 6.35) -> (-529.8504, 6.35)
  line L2559 (-529.8504, 6.35) -> (-529.8504, 9.35)
  line L2560 (-529.8504, 9.35) -> (-526.8504, 9.35)
  line L2561 (-526.8504, 9.35) -> (-526.8504, 6.35)
  line L2562 (-526.8504, 6.35) -> (-523.8504, 6.35)
  line L2563 (-523.8504, 6.35) -> (-523.8504, 9.35)
  line L2564 (-523.8504, 9.35) -> (-520.8504, 9.35)
  line L2565 (-520.8504, 9.35) -> (-520.8504, 6.35)
  line L2566 (-520.8504, 6.35) -> (-517.8504, 6.35)
  line L2567 (-517.8504, 6.35) -> (-517.8504, 9.35)
  line L2568 (-517.8504, 9.35) -> (-514.8504, 9.35)
  line L2569 (-514.8504, 9.35) -> (-514.8504, 6.35)
  line L2570 (-514.8504, 6.35) -> (-511.8504, 6.35)
  line L2571 (-511.8504, 6.35) -> (-511.8504, 9.35)
  line L2572 (-511.8504, 9.35) -> (-508.8504, 9.35)
  line L2573 (-508.8504, 9.35) -> (-508.8504, 6.35)
  line L2574 (-508.8504, 6.35) -> (-505.8504, 6.35)
  line L2575 (-505.8504, 6.35) -> (-505.8504, 9.35)
  line L2576 (-505.8504, 9.35) -> (-502.8504, 9.35)
  line L2577 (-502.8504, 9.35) -> (-502.8504, 6.35)
  line L2578 (-502.8504, 6.35) -> (-499.8504, 6.35)
  line L2579 (-499.8504, 6.35) -> (-499.8504, 9.35)
  line L2580 (-499.8504, 9.35) -> (-496.8504, 9.35)
  line L2581 (-496.8504, 9.35) -> (-496.8504, 6.35)
  line L2582 (-496.8504, 6.35) -> (-493.8504, 6.35)
  line L2583 (-493.8504, 6.35) -> (-493.8504, 9.35)
  line L2584 (-493.8504, 9.35) -> (-490.8504, 9.35)
  line L2585 (-490.8504, 9.35) -> (-490.8504, 6.35)
  line L2586 (-490.8504, 6.35) -> (-487.8504, 6.35)
  line L2587 (-487.8504, 6.35) -> (-487.8504, 9.35)
  line L2588 (-487.8504, 9.35) -> (-484.8504, 9.35)
  line L2589 (-484.8504, 9.35) -> (-484.8504, 6.35)
  line L2590 (-484.8504, 6.35) -> (-481.8504, 6.35)
  line L2591 (-481.8504, 6.35) -> (-481.8504, 9.35)
  line L2592 (-481.8504, 9.35) -> (-478.8504, 9.35)
  line L2593 (-478.8504, 9.35) -> (-478.8504, 6.35)
  line L2594 (-478.8504, 6.35) -> (-475.8504, 6.35)
  line L2595 (-475.8504, 6.35) -> (-475.8504, 9.35)
  line L2596 (-475.8504, 9.35) -> (-472.8504, 9.35)
  line L2597 (-472.8504, 9.35) -> (-472.8504, 6.35)
  line L2598 (-472.8504, 6.35) -> (-469.8504, 6.35)
  line L2599 (-469.8504, 6.35) -> (-469.8504, 9.35)
  line L2600 (-469.8504, 9.35) -> (-466.8504, 9.35)
  line L2601 (-466.8504, 9.35) -> (-466.8504, 6.35)
  line L2602 (-466.8504, 6.35) -> (-463.8504, 6.35)
  line L2603 (-463.8504, 6.35) -> (-463.8504, 9.35)
  line L2604 (-463.8504, 9.35) -> (-460.8504, 9.35)
  line L2605 (-460.8504, 9.35) -> (-460.8504, 6.35)
  line L2606 (-460.8504, 6.35) -> (-457.8504, 6.35)
  line L2607 (-457.8504, 6.35) -> (-457.8504, 9.35)
  line L2608 (-457.8504, 9.35) -> (-454.8504, 9.35)
  line L2609 (-454.8504, 9.35) -> (-454.8504, 6.35)
  line L2610 (-454.8504, 6.35) -> (-451.8504, 6.35)
  line L2611 (-451.8504, 6.35) -> (-451.8504, 9.35)
  line L2612 (-451.8504, 9.35) -> (-448.8504, 9.35)
  line L2613 (-448.8504, 9.35) -> (-448.8504, 6.35)
  line L2614 (-448.8504, 6.35) -> (-445.8504, 6.35)
  line L2615 (-445.8504, 6.35) -> (-445.8504, 9.35)
  line L2616 (-445.8504, 9.35) -> (-442.8504, 9.35)
  line L2617 (-442.8504, 9.35) -> (-442.8504, 6.35)
  line L2618 (-442.8504, 6.35) -> (-439.8504, 6.35)
  line L2619 (-439.8504, 6.35) -> (-439.8504, 9.35)
  line L2620 (-439.8504, 9.35) -> (-436.8504, 9.35)
  line L2621 (-436.8504, 9.35) -> (-436.8504, 6.35)
  line L2622 (-436.8504, 6.35) -> (-433.8504, 6.35)
  line L2623 (-433.8504, 6.35) -> (-433.8504, 9.35)
  line L2624 (-433.8504, 9.35) -> (-430.8504, 9.35)
  line L2625 (-430.8504, 9.35) -> (-430.8504, 6.35)
  line L2626 (-430.8504, 6.35) -> (-427.8504, 6.35)
  line L2627 (-427.8504, 6.35) -> (-427.8504, 9.35)
  line L2628 (-427.8504, 9.35) -> (-424.8503, 9.35)
  line L2629 (-424.8503, 9.35) -> (-424.8503, 6.35)
  line L2630 (-424.8503, 6.35) -> (-421.8503, 6.35)
  line L2631 (-421.8503, 6.35) -> (-421.8503, 9.35)
  line L2632 (-421.8503, 9.35) -> (-418.8503, 9.35)